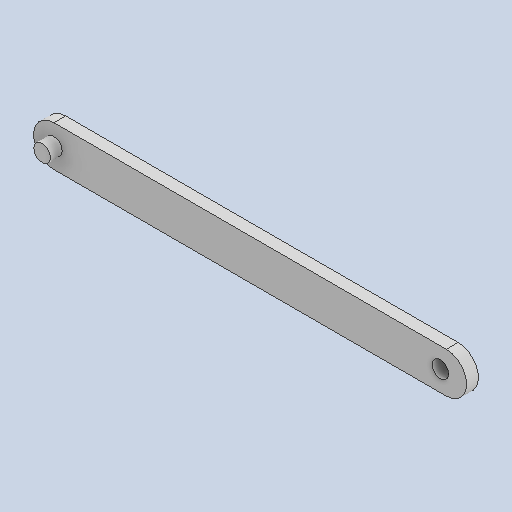
# Autodesk Inventor part: connector linkage_CPY
Saved by Autodesk Inventor 2024.1 (Build 281209000, 209)
## iProperties
Created: 2024-01-20
Part Number: connector linkage_CPY
Material: Generic
Document SubType Name: Modeling
Designer: udayk
Density: 1 g/cm^3
Appearance: Default
Author: luxsu
Autodesk Inventor part; units mm, degrees
ref_plane "YZ Plane" through (0, 0, 0) normal (1, 0, 0) x (0, 1, 0)
ref_plane "XZ Plane" through (0, 0, 0) normal (0, 1, 0) x (-1, 0, 0)
ref_plane "XY Plane" through (0, 0, 0) normal (0, 0, 1) x (1, 0, 0)
sketch "Sketch1" plane through (0, 0, 0) normal (0, 0, 1) x (1, 0, 0)
  line L0 (0, 0) -> (100, 0) construction
  line L1 (0, -5.1674) -> (100, -5.1674)
  line L2 (100, 5.1674) -> (0, 5.1674)
  arc A0 (0, 5.1674) -> (0, -5.1674) centre (0, 0) ccw
  arc A1 (100, -5.1674) -> (100, 5.1674) centre (100, 0) ccw
  point P0 (50, 0)
  dimension "d0" = 100
  constraints: 8 end point, 4 point on circle, 4 tangent, 2 centre point, 1 horizontal, 1 midpoint, 1 parallel
  measures "d0" distance of L0.end L0.start
extrude "Extrusion1" add sketch "Sketch1" along normal blind 3
sketch "Sketch2" plane through (0, 0, 3) normal (0, 0, 1) x (1, 0, 0)
  circle A0 centre (0, 0) radius 2.125
  dimension "d3" = 4.25
  constraints: 1 centre point, 1 coincident
  measures "d3" diameter of A0
extrude "Extrusion2" add sketch "Sketch2" along normal blind 3 and the other way blind 6
sketch "Sketch3" plane through (0, 0, 3) normal (0, 0, 1) x (1, 0, 0)
  circle A0 centre (140.404, 0) radius 2.125
  point P0 (0, 0)
  dimension "d8" = 4.25
  constraints: 1 centre point
  measures "d8" diameter of A0
extrude "Extrusion3" cut sketch "Sketch3" against normal blind 3
sketch "Sketch4" plane through (0, 0, 3) normal (0, 0, 1) x (1, 0, 0)
  circle A0 centre (120.4729, 0) radius 2.125
  point P0 (0, 0)
  dimension "d11" = 4.25
  constraints: 1 centre point
  measures "d11" diameter of A0
extrude "Extrusion4" cut sketch "Sketch4" against normal blind 10
sketch "Sketch5" plane through (0, 0, 3) normal (0, 0, 1) x (1, 0, 0)
  circle A0 centre (98.4795, 0) radius 2.125
  point P0 (0, 0)
  dimension "d14" = 4.25
  constraints: 1 centre point
  measures "d14" diameter of A0
extrude "Extrusion5" cut sketch "Sketch5" against normal blind 10
body "Solid1"
